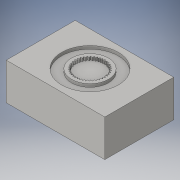
# Autodesk Inventor part: Part1
Saved by Autodesk Inventor 2016 (Build 200138000, 138)
## iProperties
Created: 2016-11-06
Part Number: Part1
Material: Generic
Document SubType Name: Modeling
Designer: adam fishburn
Density: 1 g/cm^3
Appearance: Default
Author: adam fishburn
Autodesk Inventor part; units mm, degrees
ref_plane "YZ Plane" through (0, 0, 0) normal (1, 0, 0) x (0, 1, 0)
ref_plane "XZ Plane" through (0, 0, 0) normal (0, 1, 0) x (-1, 0, 0)
ref_plane "XY Plane" through (0, 0, 0) normal (0, 0, 1) x (1, 0, 0)
sketch "Sketch1" plane through (0, 0, 0) normal (0, 1, 0) x (-1, 0, 0)
  line L0 (0, 0) -> (203.2, 0)
  line L1 (203.2, 0) -> (203.2, -142.24)
  line L2 (203.2, -142.24) -> (0, -142.24)
  line L3 (0, -142.24) -> (0, 0)
  dimension "d0" = 203.2
  dimension "d1" = 142.24
  constraints: 8 end point, 2 parallel, 1 horizontal, 1 perpendicular
  measures "d0" distance of L1.end L2.end
  measures "d1" distance of L0.end L1.end
extrude "Extrusion1" add sketch "Sketch1" along normal blind 76.2
sketch "Sketch2" plane through (0, 76.2, 0) normal (0, 1, 0) x (1, 0, 0)
  line L0 (-203.2, 0) -> (0, 0) projected
  line L1 (-203.2, 0) -> (-203.2, 71.12)
  line L2 (-203.2, 142.24) -> (-203.2, 0) projected
  line L3 (0, 0) -> (0, 142.24) projected
  line L4 (0, 0) -> (-101.6, 0)
  circle A0 centre (-101.6, 71.12) radius 38.1
  circle A1 centre (-101.6, 71.12) radius 58.42
  circle A2 centre (-101.6, 71.12) radius 31.75
  line L5 (0, 142.24) -> (-203.2, 142.24) projected
  dimension "d4" = 71.12
  dimension "d6" = 101.6
  dimension "d7" = 76.2
  dimension "d8" = 116.84
  dimension "d9" = 63.5
  dimension "d10" = 71.12
  constraints: 4 end point, 3 centre point, 2 coincident, 2 midpoint
  measures "d4" distance of L0.start L1.end
  measures "d6" distance of L0.end L4.end
  measures "d7" diameter of A0
  measures "d8" diameter of A1
  measures "d9" diameter of A2
  measures "d10" distance from line of L5 A0.centre
extrude "Extrusion2" cut sketch "Sketch2" against normal blind 6.35 contours A1
sketch "Sketch3" plane through (0, 76.2, 0) normal (0, 1, 0) x (1, 0, 0)
  line L0 (0, 0) -> (-101.6, 0)
  line L1 (-203.2, 0) -> (0, 0) projected
  line L2 (0, 142.24) -> (-203.2, 142.24) projected
  line L3 (0, 0) -> (0, 142.24) projected
  circle A0 centre (-101.5719, 71.12) radius 31.75
  line L4 (-133.3219, 71.12) -> (-129.54, 71.12) construction
  line L5 (-130.036, 73.0239) -> (-126.4684, 73.0239) construction
  line L6 (-133.3219, 71.12) -> (-130.0051, 68.7994)
  line L7 (-130.0051, 68.7994) -> (-132.8994, 65.9574)
  line L8 (-133.3219, 71.1322) -> (-130.005, 73.442)
  line L9 (-130.005, 73.442) -> (-132.8994, 76.2826)
  line L10 (-132.8994, 76.2826) -> (-129.2464, 78.0447)
  line L11 (-129.2464, 78.0447) -> (-131.6634, 81.2473)
  line L12 (-131.6634, 81.2473) -> (-127.8155, 82.305)
  line L13 (-127.8155, 82.305) -> (-129.54, 86.1483)
  line L14 (-129.54, 86.1483) -> (-125.61, 86.4823)
  line L15 (-125.61, 86.4823) -> (-126.7161, 90.5064)
  line L16 (-126.7161, 90.5064) -> (-122.6466, 90.3473)
  line L17 (-122.6466, 90.3473) -> (-123.1432, 94.4168)
  line L18 (-123.1432, 94.4168) -> (-119.1835, 93.5625)
  line L19 (-119.1835, 93.5625) -> (-119.1835, 97.5377)
  line L20 (-119.1835, 97.5377) -> (-115.486, 96.0244)
  line L21 (-115.486, 96.0244) -> (-114.8554, 99.9577)
  line L22 (-114.8554, 99.9577) -> (-111.4463, 97.8843)
  line L23 (-111.4463, 97.8843) -> (-110.657, 101.5424)
  line L24 (-110.657, 101.5424) -> (-107.6807, 98.986)
  line L25 (-107.6807, 98.986) -> (-106.2317, 102.5262)
  line L26 (-106.2317, 102.5262) -> (-103.9961, 99.5445)
  line L27 (-103.9961, 99.5445) -> (-101.6, 102.87)
  line L28 (-130.005, 68.798) -> (-132.8994, 65.9574)
  line L29 (-132.8994, 65.9574) -> (-129.2464, 64.1953)
  line L30 (-129.2464, 64.1953) -> (-131.6634, 60.9927)
  line L31 (-131.6634, 60.9927) -> (-127.8155, 59.935)
  line L32 (-127.8155, 59.935) -> (-129.54, 56.0917)
  line L33 (-129.54, 56.0917) -> (-125.61, 55.7577)
  line L34 (-125.61, 55.7577) -> (-126.7161, 51.7336)
  line L35 (-126.7161, 51.7336) -> (-122.6466, 51.8927)
  line L36 (-122.6466, 51.8927) -> (-123.1432, 47.8232)
  line L37 (-123.1432, 47.8232) -> (-119.1835, 48.6775)
  line L38 (-119.1835, 48.6775) -> (-119.1835, 44.7023)
  line L39 (-119.1835, 44.7023) -> (-115.486, 46.2156)
  line L40 (-115.486, 46.2156) -> (-114.8554, 42.2823)
  line L41 (-114.8554, 42.2823) -> (-111.4463, 44.3557)
  line L42 (-111.4463, 44.3557) -> (-110.657, 40.6976)
  line L43 (-110.657, 40.6976) -> (-107.6807, 43.254)
  line L44 (-107.6807, 43.254) -> (-106.2317, 39.7138)
  line L45 (-106.2317, 39.7138) -> (-103.9961, 42.6955)
  line L46 (-103.9961, 42.6955) -> (-101.6, 39.37)
  line L47 (-73.1943, 68.7985) -> (-70.2466, 65.9445)
  line L48 (-69.8219, 71.1322) -> (-73.1695, 73.4245)
  line L49 (-73.1695, 73.4245) -> (-70.2466, 76.2955)
  line L50 (-70.2466, 76.2955) -> (-73.9311, 78.0745)
  line L51 (-73.9311, 78.0745) -> (-71.4902, 81.2764)
  line L52 (-71.4902, 81.2764) -> (-75.3845, 82.305)
  line L53 (-75.3845, 82.305) -> (-73.6219, 86.1817)
  line L54 (-73.6219, 86.1817) -> (-77.59, 86.4823)
  line L55 (-77.59, 86.4823) -> (-76.4523, 90.5383)
  line L56 (-76.4523, 90.5383) -> (-80.5385, 90.348)
  line L57 (-80.5385, 90.348) -> (-80.038, 94.449)
  line L58 (-80.038, 94.449) -> (-84.0015, 93.5938)
  line L59 (-84.0015, 93.5938) -> (-84.0015, 97.5649)
  line L60 (-84.0015, 97.5649) -> (-87.7172, 96.0441)
  line L61 (-87.7172, 96.0441) -> (-88.3345, 99.9789)
  line L62 (-88.3345, 99.9789) -> (-91.7537, 97.8843)
  line L63 (-91.7537, 97.8843) -> (-92.5392, 101.558)
  line L64 (-92.5392, 101.558) -> (-95.5193, 98.986)
  line L65 (-95.5193, 98.986) -> (-96.9668, 102.5343)
  line L66 (-96.9668, 102.5343) -> (-99.2039, 99.5445)
  line L67 (-99.2039, 99.5445) -> (-101.6, 102.87)
  line L68 (-69.8219, 71.1322) -> (-73.195, 68.798)
  line L69 (-73.195, 68.798) -> (-70.2466, 65.9445)
  line L70 (-70.2466, 65.9445) -> (-73.9536, 64.1953)
  line L71 (-73.9536, 64.1953) -> (-71.4902, 60.9636)
  line L72 (-71.4902, 60.9636) -> (-75.3845, 59.935)
  line L73 (-75.3845, 59.935) -> (-73.6219, 56.0583)
  line L74 (-73.6219, 56.0583) -> (-77.59, 55.7577)
  line L75 (-76.4527, 51.701) -> (-80.5534, 51.8927)
  line L76 (-77.59, 55.7577) -> (-76.4527, 51.701)
  line L77 (-80.5534, 51.8927) -> (-80.0351, 47.7913)
  line L78 (-80.0351, 47.7913) -> (-84.0015, 48.6742)
  line L79 (-84.0015, 48.6742) -> (-84.0015, 44.6736)
  line L80 (-84.0015, 44.6736) -> (-87.714, 46.2156)
  line L81 (-87.714, 46.2156) -> (-88.3345, 42.2611)
  line L82 (-88.3345, 42.2611) -> (-91.7537, 44.3557)
  line L83 (-91.7537, 44.3557) -> (-92.5392, 40.682)
  line L84 (-92.5392, 40.682) -> (-95.5193, 43.254)
  line L85 (-95.5193, 43.254) -> (-96.9683, 39.7055)
  line L86 (-96.9683, 39.7055) -> (-99.2039, 42.6955)
  line L87 (-99.2039, 42.6955) -> (-101.6, 39.37)
  line L88 (-133.3219, 71.1322) -> (-130.005, 68.798)
  line L89 (-130.005, 68.798) -> (-132.8994, 65.9574)
  line L90 (-132.8994, 65.9574) -> (-129.2464, 64.1953)
  line L91 (-129.2464, 64.1953) -> (-131.6634, 60.9927)
  line L92 (-131.6634, 60.9927) -> (-127.8155, 59.935)
  line L93 (-127.8155, 59.935) -> (-129.54, 56.0917)
  line L94 (-126.7161, 51.7336) -> (-122.6466, 51.8927)
  line L95 (-122.6466, 51.8927) -> (-123.1432, 47.8232)
  line L96 (-123.1432, 47.8232) -> (-119.1835, 48.6775)
  line L97 (-119.1835, 48.6775) -> (-119.1835, 44.7023)
  line L98 (-119.1835, 44.7023) -> (-115.486, 46.2156)
  line L99 (-115.486, 46.2156) -> (-114.8554, 42.2823)
  line L100 (-114.8554, 42.2823) -> (-111.4463, 44.3557)
  line L101 (-111.4463, 44.3557) -> (-110.657, 40.6976)
  line L102 (-107.6807, 43.254) -> (-110.657, 40.6976)
  line L103 (-107.6807, 43.254) -> (-106.2317, 39.7138)
  line L104 (-106.2317, 39.7138) -> (-103.9961, 42.6955)
  line L105 (-103.9961, 42.6955) -> (-101.6, 39.37)
  line L106 (-101.6, 39.37) -> (-99.2039, 42.6955)
  line L107 (-99.2039, 42.6955) -> (-96.9683, 39.7055)
  line L108 (-96.9683, 39.7055) -> (-95.5193, 43.254)
  line L109 (-95.5193, 43.254) -> (-92.5392, 40.682)
  line L110 (-92.5392, 40.682) -> (-91.7537, 44.3557)
  line L111 (-91.7537, 44.3557) -> (-88.3345, 42.2611)
  line L112 (-129.2464, 78.0447) -> (-131.6634, 81.2473)
  line L113 (-131.6634, 81.2473) -> (-127.8155, 82.305)
  line L114 (-129.54, 86.1483) -> (-127.8155, 82.305)
  line L115 (-129.54, 86.1483) -> (-125.61, 86.4823)
  line L116 (-125.61, 86.4823) -> (-126.7161, 90.5064)
  line L117 (-71.4902, 81.2764) -> (-73.9311, 78.0745)
  line L118 (-73.9311, 78.0745) -> (-70.2466, 76.2955)
  line L119 (-70.2466, 76.2955) -> (-73.1695, 73.4245)
  line L120 (-73.1695, 73.4245) -> (-69.8219, 71.1322)
  line L121 (-69.8219, 71.1322) -> (-73.1943, 68.7985)
  line L122 (-73.1943, 68.7985) -> (-70.2466, 65.9445)
  line L123 (-70.2466, 65.9445) -> (-73.9536, 64.1953)
  line L124 (-73.9536, 64.1953) -> (-71.4902, 60.9636)
  line L125 (-71.4902, 60.9636) -> (-75.3845, 59.935)
  line L126 (-75.3845, 59.935) -> (-73.6219, 56.0583)
  line L127 (-75.3845, 59.935) -> (-73.6219, 56.0583)
  line L128 (-73.6219, 56.0583) -> (-77.59, 55.7577)
  line L129 (-70.2466, 65.9445) -> (-73.1943, 68.7985)
  line L130 (-73.1943, 68.7985) -> (-69.8219, 71.1322)
  line L131 (-69.8219, 71.1322) -> (-73.1695, 73.4245)
  line L132 (-73.1695, 73.4245) -> (-70.2466, 76.2955)
  line L133 (-70.2466, 76.2955) -> (-73.9311, 78.0745)
  line L134 (-71.4902, 60.9636) -> (-73.9536, 64.1953)
  line L135 (-73.9536, 64.1953) -> (-70.2466, 65.9445)
  line L136 (-70.2466, 65.9445) -> (-73.1943, 68.7985)
  line L137 (-73.1943, 68.7985) -> (-70.2466, 65.9445)
  line L138 (-73.1943, 68.7985) -> (-69.8219, 71.1322)
  line L139 (-69.8219, 71.1322) -> (-73.1695, 73.4245)
  line L140 (-73.1695, 73.4245) -> (-70.2466, 76.2955)
  line L141 (-70.2466, 76.2955) -> (-73.9311, 78.0745)
  line L142 (-69.8219, 71.1322) -> (-73.1695, 73.4245)
  line L143 (-71.4902, 81.2764) -> (-75.3845, 82.305)
  line L144 (-75.3845, 82.305) -> (-73.6219, 86.1817)
  line L145 (-73.6219, 86.1817) -> (-77.59, 86.4823)
  line L146 (-77.59, 86.4823) -> (-76.4523, 90.5383)
  line L147 (-73.6219, 86.1817) -> (-77.59, 86.4823)
  line L148 (-80.5385, 90.348) -> (-76.4523, 90.5383)
  line L149 (-71.4902, 81.2764) -> (-73.9311, 78.0745)
  line L150 (-131.6634, 81.2473) -> (-127.8155, 82.305)
  line L151 (-127.8155, 82.305) -> (-129.54, 86.1483)
  line L152 (-129.54, 86.1483) -> (-127.8155, 82.305)
  line L153 (-129.54, 86.1483) -> (-125.61, 86.4823)
  line L154 (-125.61, 86.4823) -> (-126.7161, 90.5064)
  line L155 (-126.7161, 90.5064) -> (-122.6466, 90.3473)
  line L156 (-122.6466, 90.3473) -> (-123.1432, 94.4168)
  line L157 (-123.1432, 94.4168) -> (-122.6466, 90.3473)
  line L158 (-123.1432, 94.4168) -> (-119.1835, 93.5625)
  line L159 (-119.1835, 93.5625) -> (-119.1835, 97.5377)
  line L160 (-119.1835, 97.5377) -> (-115.486, 96.0244)
  line L161 (-115.486, 96.0244) -> (-114.8554, 99.9577)
  line L162 (-114.8554, 99.9577) -> (-111.4463, 97.8843)
  dimension "d13" = 63.5
  dimension "d27" = 69.832
  dimension "d28" = 70.214
  dimension "d29" = 79.316
  dimension "d30" = 78.709
  dimension "d31" = 77.824
  constraints: 320 end point, 42 collinear, 3 perpendicular, 3 vertical, 2 horizontal, 2 point on line, 1 midpoint, 32 other
  measures "d27" angle of L8 L6
  measures "d28" angle of L10 L9
  measures "d29" angle of L9 L8
  measures "d30" angle of L11 L10
  measures "d31" angle of L19 L18
extrude "Extrusion3" cut sketch "Sketch3" against normal blind 6.35 contours L68 L47 L70 L71 L72 L73 L74 L76 L75 L77 L78 L79 L80 L81 L82 L83 L84 L85 L86 L87 L46 L45 L44 L43 L42 L41 L40 L39 L38 L37 L36 L35 L34 L33 L32 L31 L30 L29 L7 L88 L8 L9 L10 L11 L12 L13 L14 L15 L16 L17 L18 L19 L20 L21 L22 L23 L24 L25 L26 L27 L67 L66 L65 L64 L63 L62 L61 L60 L59 L58 L57 L56 L55 L54 L53 L52 L51 L50 L49 L48 | A0 L88 L6
body "Solid1"
